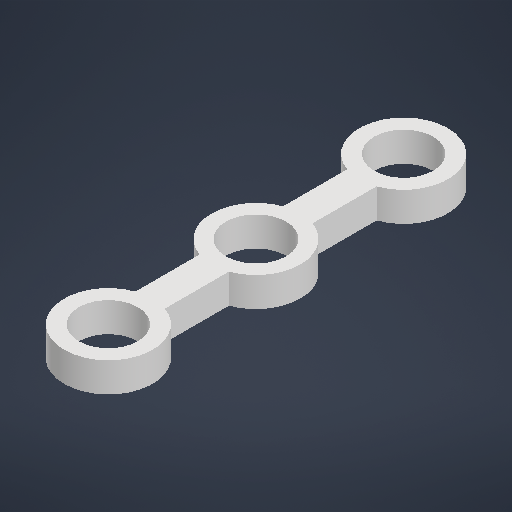
# Autodesk Inventor part: Pillar_side
Saved by Autodesk Inventor 2026 (Build 300175050, 175E)
## iProperties
Created: 2026-06-21
Part Number: Pillar_side
Material: Generic
Document SubType Name: Modeling
Designer: sniel
Density: 1 g/cm^3
Appearance: Default
Author: sniel
Autodesk Inventor part; units mm, degrees
ref_plane "YZ Plane" through (0, 0, 0) normal (1, 0, 0) x (0, 1, 0)
ref_plane "XZ Plane" through (0, 0, 0) normal (0, 1, 0) x (-1, 0, 0)
ref_plane "XY Plane" through (0, 0, 0) normal (0, 0, 1) x (1, 0, 0)
sketch "Sketch1" plane through (0, 0, 0) normal (0, 1, 0) x (-1, 0, 0)
  circle A0 centre (0, 0) radius 5
  circle A1 centre (0, 0) radius 7.5
  line L0 (-2.5, -5) -> (2.5, -5)
  line L1 (2.5, -5) -> (2.5, -10)
  line L2 (2.5, -10) -> (-2.5, -10)
  line L3 (-2.5, -10) -> (-2.5, -5)
  line L4 (-2.5, -5) -> (2.5, -10) construction
  line L5 (2.5, -5) -> (-2.5, -10) construction
  line L6 (0, 0) -> (0, -50)
  line L7 (0, -25) -> (5, -25)
  circle A2 centre (0, -50) radius 5
  circle A3 centre (0, -50) radius 7.5
  line L8 (-2.5, -45) -> (2.5, -45)
  line L9 (2.5, -45) -> (2.5, -40)
  line L10 (2.5, -40) -> (-2.5, -40)
  line L11 (-2.5, -40) -> (-2.5, -45)
  line L12 (-2.5, -45) -> (2.5, -40) construction
  line L13 (2.5, -45) -> (-2.5, -40) construction
  line L14 (2.5, -7.0711) -> (2.5, -42.9289)
  line L15 (-2.5, -42.9289) -> (-2.5, -7.0711)
  circle A4 centre (0, -25) radius 5
  circle A5 centre (0, -25) radius 7.5
  circle A6 centre (0, -25) radius 5.1
  point P0 (0, -7.5)
  point P1 (0, -42.5)
  point P2 (-2.5, -17.9289)
  point P3 (-2.5, -32.0711)
  point P4 (2.5, -32.0711)
  point P5 (2.5, -17.9289)
  dimension "d0" = 10
  dimension "d1" = 15
  dimension "d2" = 5
  dimension "d3" = 5
  dimension "d4" = 50
  dimension "d7" = 10
  dimension "d8" = 15
  dimension "d9" = 10.2
  constraints: 32 end point, 7 centre point, 7 coincident, 7 symmetric about line, 6 point on circle, 4 point on line, 3 midpoint, 2 horizontal, 2 parallel, 1 perpendicular, 1 vertical, 2 other
  measures "d0" diameter of A0
  measures "d1" diameter of A1
  measures "d2" distance of L1.end L2.end
  measures "d3" distance of L0.end L1.end
  measures "d4" distance of L6.start L6.end
  measures "d7" diameter of A4
  measures "d8" diameter of A5
  measures "d9" diameter of A6
extrude "Extrusion1" add sketch "Sketch1" along normal blind 5 contours L0 L3 A1 L1 | L0 L1 A1 L6 | L6 A1 L3 L0 | L6 L2 L3 A1 | A1 L1 L2 L6 | L6 A5 L15 L2 | L2 L14 A5 L6 | A5 L14 A6 L6 | L6 A6 L15 A5 | L15 A6 A5 | A5 L14 A6 | A5 L6 L10 L15 | L15 A6 L6 A5 | L10 L6 A3 L11 | A5 L14 L10 L6 | L6 A6 L14 A5 | L10 L9 A3 L6 | L11 L8 L9 A3 | A3 L6 L8 L11 | A3 L9 L8 L6
body "Solid1"
